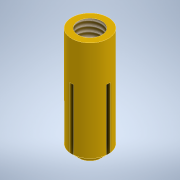
# Autodesk Inventor part: clamping_insert
Saved by Autodesk Inventor 2021 (Build 250183000, 183)
## iProperties
Created: 2022-06-12
Part Number: clamping_insert
Material: Generic
Document SubType Name: Modeling
Designer: lenna
Density: 1 g/cm^3
Appearance: Gold
Author: lenna
Autodesk Inventor part; units mm, degrees
ref_plane "YZ Plane" through (0, 0, 0) normal (1, 0, 0) x (0, 1, 0)
ref_plane "XZ Plane" through (0, 0, 0) normal (0, 1, 0) x (-1, 0, 0)
ref_plane "XY Plane" through (0, 0, 0) normal (0, 0, 1) x (1, 0, 0)
sketch "Sketch1" plane through (0, 0, 0) normal (0, 1, 0) x (-1, 0, 0)
  circle A0 centre (0, 0) radius 3.75
  dimension "d0" = 7.5
  constraints: 1 centre point, 1 coincident
  measures "d0" diameter of A0
extrude "Extrusion1" add sketch "Sketch1" along normal blind 22
sketch "Sketch2" plane through (0, 22, 0) normal (0, 1, 0) x (1, 0, 0)
  circle A0 centre (0, 0) radius 3.75 projected
  constraints: 1 coincident
hole "Hole1" at (0, 22, 0) direction (0, -1, 0) diameter 4.917 depth 20 tip angle 118 thread size "M6x1" class "6H" standard "ISO Metric profile"
chamfer "Chamfer1" distance 1.5 angle 45 1 edges at (3.75, 0, 0)
sketch "Sketch4" plane through (0, 0, 0) normal (1, 0, 0) x (0, 1, 0)
  line L0 (0, -2.25) -> (0, 2.25) projected
  line L1 (0, -0.4) -> (14, -0.4)
  line L2 (14, -0.4) -> (14, 0.4)
  line L3 (14, 0.4) -> (0, 0.4)
  line L4 (0, 0.4) -> (0, -0.4)
  point P0 (0, 0)
  point P1 (0, 0.4)
  dimension "d19" = 0.8
  dimension "d20" = 0.4
  dimension "d21" = 14
  constraints: 8 end point, 2 parallel, 1 horizontal, 1 perpendicular, 1 point on line
  measures "d19" distance between parallel lines of L3 L1
  measures "d20" distance from line of point (0, 0) L1
  measures "d21" distance between parallel lines of L0 L2
sketch "Sketch5" plane through (0, 0, 0) normal (0, -1, 0) x (1, 0, 0)
  circle A0 centre (0, 0) radius 1.5
  dimension "d16" = 3
  constraints: 1 centre point, 1 coincident
  measures "d16" diameter of A0
extrude "Extrusion3" cut sketch "Sketch5" against normal through all
extrude "Extrusion4" cut sketch "Sketch4" along normal through all both and the other way through all
pattern_circular "Circular Pattern1" count 4 over 360 about axis through (0, 0, 0) along (0, 1, 0) of "Extrusion4"
equation "\"d20\" = 0.5 * d19"
body "Solid1"
